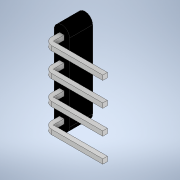
# Autodesk Inventor part: Conector
Saved by Autodesk Inventor 2021 (Build 250183000, 183)
## iProperties
Created: 2021-06-10
Part Number: Conector
Material: Genérico
Document SubType Name: Modeling
Designer: rubia
Density: 1 g/cm^3
Appearance: Padrão
Author: rubia
Autodesk Inventor part; units mm, degrees
ref_plane "YZ Plane" through (0, 0, 0) normal (1, 0, 0) x (0, 1, 0)
ref_plane "XZ Plane" through (0, 0, 0) normal (0, 1, 0) x (-1, 0, 0)
ref_plane "XY Plane" through (0, 0, 0) normal (0, 0, 1) x (1, 0, 0)
sketch "Esboço1" plane through (0, 0, 0) normal (0, 0, 1) x (1, 0, 0)
  line L0 (0, 0) -> (0, 10) construction
  line L1 (1, 0) -> (1, 10)
  line L2 (-1, 10) -> (-1, 0)
  arc A0 (-1, 0) -> (1, 0) centre (0, 0) ccw
  arc A1 (1, 10) -> (-1, 10) centre (0, 10) ccw
  point P0 (0, 5)
  dimension "d0" = 10
  dimension "d1" = 2
  constraints: 8 end point, 4 point on circle, 4 tangent, 2 centre point, 1 midpoint, 1 parallel, 1 vertical
  measures "d0" distance of L0.start L0.end
  measures "d1" diameter of A1
extrude "Extrusão1" add sketch "Esboço1" along normal blind 3
sketch "Esboço2" plane through (0, 0, 3) normal (0, 0, 1) x (1, 0, 0)
  arc A0 (1, 10) -> (-1, 10) centre (0, 10) ccw construction
  arc A1 (-1, 0) -> (1, 0) centre (0, 0) ccw construction
  line L0 (0, 10) -> (0, 0) construction
  line L1 (-1, 10) -> (-1, 0) construction
  line L2 (-1, 0) -> (1, 0) construction
  line L3 (0.3, 0) -> (-0.3, 0)
  line L4 (-0.3, 0) -> (-0.3, 0.6)
  line L5 (-0.3, 0.6) -> (0.3, 0.6)
  line L6 (0.3, 0.6) -> (0.3, 0)
  dimension "d4" = 0.6
  dimension "d5" = 0.6
  dimension "d6" = 0.6
  dimension "d7" = 0.3
  constraints: 12 end point, 3 perpendicular, 2 point on line, 1 vertical
  measures "d4" distance of L3.start L3.end
  measures "d5" distance of L3.end L4.end
  measures "d6" distance of L4.end L5.end
  measures "d7" distance from line of L4 point (0, 0)
extrude "Extrusão2" add sketch "Esboço2" along normal blind 2
sketch "Esboço3" plane through (0, 0, 5) normal (0, 0, 1) x (1, 0, 0)
  line L0 (0.3, 0) -> (-0.3, 0) projected
  line L1 (-0.3, 0.6) -> (0.3, 0.6) projected
  line L2 (0.3, 0.6) -> (0.3, 0)
  line L3 (0.3, 0.6) -> (0.3, 0) projected
  line L4 (0.3, 0.6) -> (7.3, 0.6)
  line L5 (7.3, 0.6) -> (7.3, 0)
  line L6 (7.3, 0) -> (0.3, 0)
  line L7 (0.3, 0) -> (0.3, 0.6)
  point P0 (0, 0)
  dimension "d13" = 7
  constraints: 10 end point, 2 perpendicular, 1 collinear, 1 horizontal
  measures "d13" distance of L1.end L4.end
extrude "Extrusão3" add sketch "Esboço3" against normal blind 0.6
fillet "Arredondamento1" radius 1 1 edges at (-0.3, 0.3, 5)
pattern_linear "Padrão retangular1" count 4 spacing 3.1333 along (0, 1, 0) of "Extrusão3", "Arredondamento1", "Extrusão2"
